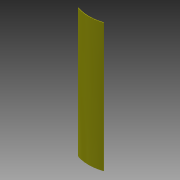
# Autodesk Inventor part: Antenna
Saved by Autodesk Inventor 2015 SP1 (Build 190203100, 203)
## iProperties
Created: 2015-06-22
Part Number: Antenna
Material: Generic
Document SubType Name: Modeling
Designer: Kartikye
Density: 1 g/cm^3
Appearance: Default
Author: Kartikye
Autodesk Inventor part; units mm, degrees
ref_plane "YZ Plane" through (0, 0, 0) normal (1, 0, 0) x (0, 1, 0)
ref_plane "XZ Plane" through (0, 0, 0) normal (0, 1, 0) x (-1, 0, 0)
ref_plane "XY Plane" through (0, 0, 0) normal (0, 0, 1) x (1, 0, 0)
sketch "Sketch2" plane through (0, 0, 0) normal (0, 0, 1) x (1, 0, 0)
  arc A0 (0, 10.7251) -> (15, 10.7251) centre (7.5, 32.25) ccw
  arc A1 (0, 10.4751) -> (15, 10.4751) centre (7.5, 32) ccw
  line L0 (0, 10.7251) -> (0, 10.4751)
  line L1 (15, 10.7251) -> (15, 10.4751)
  point P0 (0, 0)
  dimension "d0" = 15
  dimension "d1" = 15
  dimension "d2" = 0.25
  constraints: 4 end point, 4 point on circle, 2 centre point, 1 parallel, 1 vertical
  measures "d0" distance of L0.start L1.start
  measures "d1" distance of L0.end L1.end
  measures "d2" distance of A1.centre A0.centre
extrude "Extrusion1" add sketch "Sketch2" along normal blind 75
body "Solid1"
